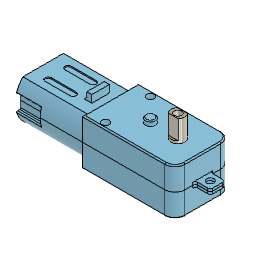
3802 TT Motor Metal Gear (Autodesk Fusion 360 design; units mm, degrees)
Autodesk Fusion 360 part; units mm, degrees
sketch "Sketch1" plane through (0, 0, 0) normal (0, 0, 1) x (1, 0, 0)
  circle A0 centre (0, 0) radius 2.7
  line L0 (-1.9666, 1.85) -> (1.9666, 1.85)
  line L1 (0, 0) -> (10, 0) construction
  line L2 (-1.9666, -1.85) -> (1.9666, -1.85)
  line L3 (-27, 11.2) -> (10, 11.2)
  line L4 (10, 11.2) -> (10, -11.2)
  line L5 (10, -11.2) -> (-27, -11.2)
  line L6 (-27, -11.2) -> (-27, 11.2)
  circle A1 centre (-20, 9) radius 1.5
  circle A2 centre (-11, 0) radius 2
  circle A3 centre (-20, -9) radius 1.5
  dimension "d1" = 5.4
  dimension "d2" = 1.85
  dimension "d3" = 22.4
  dimension "d4" = 10
  dimension "d5" = 37
  dimension "d6" = 3
  dimension "d7" = 20
  dimension "d8" = 9
  dimension "d9" = 4
  dimension "d10" = 9
  constraint coincident A0.centre L1.start
  constraint coincident A0 L0.start
  constraint coincident A0 L0.end
  constraint horizontal L0
  constraint horizontal L1
  constraint symmetric L0.start L1 L2.start
  constraint symmetric L0.end L1 L2.end
  constraint horizontal L3
  constraint vertical L4
  constraint horizontal L5
  constraint vertical L6
  constraint midpoint L1.end L4
  constraint coincident L1 A2.centre
  constraint symmetric L1 A1 A3
  measures "d1" diameter of A0
  measures "d2" distance of A0.centre L0
  measures "d3" distance of L3.end L4.end
  measures "d4" distance of A0.centre L1.end
  measures "d5" distance of L3.start L3.end
  measures "d6" diameter of A1
  measures "d7" horizontal distance of A0.centre A1.centre
  measures "d8" vertical distance of A0.centre A1.centre
  measures "d9" diameter of A2
  measures "d10" horizontal distance of A1.centre A2.centre
  measures "d45" distance of A0.centre
extrude "Extrude1" add sketch "Sketch1" against normal blind 18.6 contours A0 L0 L2 | A0 L0 | A0 L2 | L3 L4 L5 L6 | A2 makes body 1
ref_plane "WorkPlane1" through (-8.5, 0, -9.3) normal (0, 0, 1) x (1, 0, 0)
sketch "Sketch2" plane through (-8.5, 0, -9.3) normal (0, 0, 1) x (1, 0, 0)
  line L0 (18.5, 11.2) -> (18.5, -11.2)
  line L1 (18.5, -3) -> (24.5, -3)
  line L2 (24.5, -3) -> (24.5, 3)
  line L3 (24.5, 3) -> (18.5, 3)
  line L4 (18.5, 3) -> (18.5, -3)
  line L5 (24.5, 0) -> (18.5, 0) construction
  circle A0 centre (21.5, 0) radius 1.5
  dimension "d23" = 6
  dimension "d24" = 6
  dimension "d25" = 3
  constraint horizontal L1
  constraint vertical L2
  constraint horizontal L3
  constraint vertical L4
  constraint midpoint L0 L4
  constraint midpoint L2 L5.start
  constraint midpoint L0 L5.end
  constraint coincident L5 A0.centre
  constraint midpoint L5 A0.centre
  measures "d23" distance of L1.start L1.end
  measures "d24" distance of L1.start L3.end
  measures "d25" diameter of A0
extrude "Extrude2" add sketch "Sketch1" along normal blind 8.7 separate body contours A0 L0 L2 makes body 2
extrude "Extrude3" add sketch "Sketch1" along normal blind 1 contours A0 L0 | A0 L2 bodies 2
extrude "Extrude4" add sketch "Sketch1" along normal blind 1.92 contours A2 bodies 1 2
chamfer "Chamfer1" distance 0.4 angle 45 1 edges at (-12.8647, -0.7232, 1.92) on bodies 1
sketch "Sketch3" plane through (-27, 0, 0) normal (-1, 0, 0) x (0, -1, 0)
  line L0 (11.2, 0) -> (-11.2, 0)
  line L1 (-11.2, 0) -> (-11.2, -18.6)
  line L2 (-11.2, -18.6) -> (11.2, -18.6)
  line L3 (11.2, -18.6) -> (11.2, 0)
  line L4 (0, 0) -> (0, -18.6) construction
  circle A0 centre (0, -9.3) radius 11.2
  line L5 (-11.2, -1.6) -> (11.2, -1.6)
  dimension "d30" = 17
  constraint coincident L4.start origin
  constraint midpoint L2 L4.end
  constraint midpoint L4 A0.centre
  constraint tangent L3 A0
  constraint coincident L1 L5.start
  constraint coincident L3 L5.end
  constraint perpendicular L3 L5
  measures "d30" distance of L2 L5
extrude "Extrude6" add sketch "Sketch3" along normal blind 27 contours L2 A0 L5 bodies 1
fillet "Fillet1" radius 4 2 edges at (10, -11.2, -9.3) (10, 11.2, -9.3) on bodies 1
fillet "Fillet2" radius 0.5 13 edges at (-27, 0, 0) (-10.5, 11.2, 0) (8.8284, 10.0284, 0) (10, 0, 0) (8.8284, -10.0284, 0) (-10.5, -11.2, 0) (-10.5, 11.2, -18.6) (8.8284, 10.0284, -18.6) (10, 0, -18.6) (8.8284, -10.0284, -18.6) (-10.5, -11.2, -18.6) (-27, -8.7205, -18.6) (-27, 8.7205, -18.6) on bodies 1
extrude "Extrude5" add sketch "Sketch2" along normal mid plane 2 bodies 2 1
fillet "Fillet3" radius 1 4 edges at (10, -3, -9.3) (10, 3, -9.3) (16, -3, -9.3) (16, 3, -9.3) on bodies 1
sketch "Sketch5" plane through (-54, 0, 0) normal (-1, 0, 0) x (0, -1, 0)
  arc A0 (-8.1333, -1.6) -> (-6.241, -18.6) centre (0, -9.3) ccw
  line L0 (-6.241, -18.6) -> (6.241, -18.6)
  arc A1 (6.241, -18.6) -> (8.1333, -1.6) centre (0, -9.3) ccw
  line L1 (8.1333, -1.6) -> (-8.1333, -1.6)
  line L2 (-14, -6.3) -> (-9, -6.3)
  line L3 (-9, -6.3) -> (-9, -12.3)
  line L4 (-9, -12.3) -> (-14, -12.3)
  line L5 (-14, -12.3) -> (-14, -6.3)
  line L6 (-9, -9.3) -> (0, -9.3) construction
  circle A2 centre (0, -9.3) radius 4
  line L7 (-2.6458, -6.3) -> (2.6458, -6.3)
  circle A3 centre (0, -9.3) radius 1
  dimension "d43" = 5
  dimension "d44" = 6
  dimension "d45" = 9
  dimension "d50" = 8
  dimension "d51" = 3
  dimension "d55" = 2
  constraint horizontal L2
  constraint vertical L3
  constraint horizontal L4
  constraint vertical L5
  constraint midpoint L3 L6.start
  constraint coincident A0.centre A1.centre
  constraint horizontal L6
  constraint concentric A0 A2
  constraint coincident A2 L7.start
  constraint coincident A2 L7.end
  constraint horizontal L7
  constraint concentric A0 A3
  measures "d43" distance of L2.start L2.end
  measures "d44" distance of L2.start L4.end
  measures "d45" distance of L6.start A0.centre
  measures "d50" diameter of A2
  measures "d51" distance of A0.centre L7
  measures "d55" diameter of A3
extrude "Extrude9" cut sketch "Sketch5" against normal blind 10 contours A0 L2 L3 L4 bodies 1
mirror "Mirror2" about plane through (0, 0, 0) normal (0, 1, 0) of "Extrude9"
fillet "Fillet4" radius 0.4 8 edges at (-49, 10.7907, -6.3) (-49, 10.7907, -12.3) (-49, 9, -12.3) (-49, 9, -6.3) (-49, -10.7907, -12.3) (-49, -9, -12.3) (-49, -9, -6.3) (-49, -10.7907, -6.3) on bodies 1
split "Split1" by plane through (-8.5, 0, -9.3) normal (0, 0, 1) bodies 2 1 makes body 3 at (3.3333, 0, 0)
sketch "Sketch4" plane through (0, 0, -1.6) normal (0, 0, 1) x (-1, 0, 0)
  line L0 (38, -5.25) -> (48, -5.25)
  arc A0 (48, -5.25) -> (48, -2.75) centre (48, -4) ccw
  line L1 (48, -2.75) -> (38, -2.75)
  arc A1 (38, -2.75) -> (38, -5.25) centre (38, -4) ccw
  line L2 (38, -4) -> (48, -4) construction
  line L3 (0, 0) -> (55.2044, 0) construction
  line L4 (38, 5.25) -> (48, 5.25)
  arc A2 (48, 2.75) -> (48, 5.25) centre (48, 4) ccw
  line L5 (48, 2.75) -> (38, 2.75)
  arc A3 (38, 5.25) -> (38, 2.75) centre (38, 4) ccw
  dimension "d33" = 2.5
  dimension "d34" = 4
  dimension "d35" = 10
  dimension "d36" = 38
  constraint tangent L0 A0
  constraint tangent A0 L1
  constraint parallel L0 L1
  constraint tangent L1 A1
  constraint tangent L0 A1
  constraint horizontal L2
  constraint coincident L3.start origin
  constraint parallel L1 L3
  constraint symmetric L0.start L3 L4.start
  constraint symmetric L0.end L3 L4.end
  constraint symmetric A0.end L3 A2.start
  constraint symmetric L1.end L3 L5.end
  constraint symmetric A0 L3 A2
  constraint symmetric A1 L3 A3
  measures "d33" diameter of A0
  measures "d34" distance of L2 L3
  measures "d35" distance of A1.centre A0.centre
  measures "d36" horizontal distance of L3.start A1.centre
extrude "Extrude7" cut sketch "Sketch4" against normal blind 0.5 bodies 3
extrude "Extrude8" cut sketch "Sketch4" along normal blind 0.5 from surface at -17 bodies 1
extrude "Extrude10" add sketch "Sketch5" along normal blind 1 separate body contours A2 L7 | A3 picked at (0.0249, -6.9676) makes body 4
fillet "Fillet5" radius 0.3 2 edges at (-55, 0, -6.3) (-55, 0, -13.3) on bodies 4
extrude "Extrude11" add sketch "Sketch5" along normal blind 1 from surface at 1 contours A3 bodies 4
fillet "Fillet6" radius 0.5 1 edges at (-56, 0.9323, -9.6616) on bodies 4
sketch "Sketch6" plane through (0, 0, -1.6) normal (0, 0, 1) x (-1, 0, 0)
  line L0 (27, -8.1333) -> (27, 8.1333)
  line L1 (31, -3.5) -> (33, -3.5)
  line L2 (33, -3.5) -> (33, 3.5)
  line L3 (33, 3.5) -> (31, 3.5)
  line L4 (31, 3.5) -> (31, -3.5)
  line L5 (31, 0) -> (27, 0) construction
  dimension "d60" = 7
  dimension "d61" = 2
  dimension "d62" = 4
  constraint horizontal L1
  constraint vertical L2
  constraint horizontal L3
  constraint vertical L4
  constraint midpoint L4 L5.start
  constraint midpoint L0 L5.end
  constraint horizontal L5
  measures "d60" distance of L1.start L3.end
  measures "d61" distance of L1.start L1.end
  measures "d62" distance of L5.start L5.end
extrude "Extrude12" add sketch "Sketch6" along normal blind 3 bodies 3
chamfer "Chamfer2" distance 1 angle 45 1 edges at (-33, 0, -1.6) on bodies 3
extrude "Extrude13" add sketch "Sketch6" against normal blind 3 from surface at -17 bodies 1
chamfer "Chamfer3" distance 1 angle 45 1 edges at (-33, 0, -18.6) on bodies 1
sketch "Sketch7" plane through (0, 0, 8.7) normal (0, 0, 1) x (-1, 0, 0)
  circle A0 centre (0, 0) radius 1.5
  dimension "d70" = 3
  dimension "d72" = 0
  constraint coincident A0.centre origin
  measures "d70" diameter of A0
extrude "Extrude14" cut sketch "Sketch7" against normal blind 6.5 bodies 2
equation "d2 = ( 3.7 / 2 ) * 1 mm"
